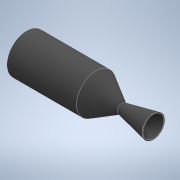
# Autodesk Inventor part: ESBOÇO 0.1 DO CAD DO MOTOR
Saved by Autodesk Inventor 2021 (Build 250183000, 183)
## iProperties
Created: 2021-01-21
Part Number: ESBOÇO 0.1 DO CAD DO MOTOR
Material: Steel AISI316
Document SubType Name: Modeling
Designer: jjunn
Mass: 349.712 g
Surface Area: 2337.95 cm^2
Volume: 349.712 cm^3
Density: 7870 g/cm^3
Appearance: Stainless Steel AISI 316
Author: jjunn
Autodesk Inventor part; units mm, degrees
ref_plane "YZ Plane" through (0, 0, 0) normal (1, 0, 0) x (0, 1, 0)
ref_plane "XZ Plane" through (0, 0, 0) normal (0, 1, 0) x (-1, 0, 0)
ref_plane "XY Plane" through (0, 0, 0) normal (0, 0, 1) x (1, 0, 0)
sketch "Sketch1" plane through (0, 0, 0) normal (0, 0, 1) x (1, 0, 0)
  line L0 (203, 55.5) -> (0, 55.5)
  line L1 (0, 55.5) -> (0, 0)
  line L2 (203, 55.5) -> (280.1, 10.9863)
  line L3 (280.1, 10.9863) -> (374.0063, 30.9467)
  line L4 (-3, 0) -> (-3, 58.5)
  line L5 (-3, 58.5) -> (203.8038, 58.5)
  line L6 (203.8038, 58.5) -> (280.6027, 14.1602)
  line L7 (280.6027, 14.1602) -> (374.0063, 34.0137)
  line L8 (-3, 0) -> (0, 0)
  line L9 (374.0063, 34.0137) -> (374.0063, 30.9467)
  line L10 (-78.4013, 0) -> (449.4075, 0) projected
  dimension "d11" = 3
  constraints: 20 end point, 1 horizontal, 1 perpendicular, 3 other
  measures "d11" distance between parallel lines of L0 L5
revolve "Revolution1" add sketch "Sketch1" angle 360 about axis through (-10, 0, 0) along (1, 0, 0)
body "Solid1"
